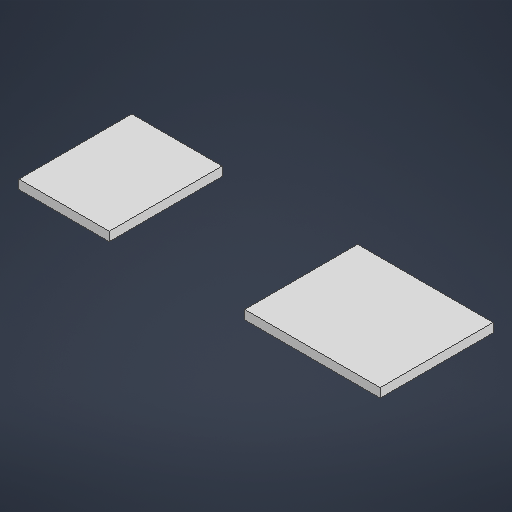
# Autodesk Inventor part: Krytka
Saved by Autodesk Inventor 2026.2 (Build 302298000, 298)
## iProperties
Created: 2026-04-16
Part Number: Krytka
Material: Všeobecné
Document SubType Name: Modeling
Designer: cerna
Density: 1 g/cm^3
Appearance: Výchozí
Author: cerna
Autodesk Inventor part; units mm, degrees
ref_plane "YZ Plane" through (0, 0, 0) normal (1, 0, 0) x (0, 1, 0)
ref_plane "XZ Plane" through (0, 0, 0) normal (0, 1, 0) x (-1, 0, 0)
ref_plane "XY Plane" through (0, 0, 0) normal (0, 0, 1) x (1, 0, 0)
sketch "Náčrt1" plane through (0, 0, 0) normal (0, 1, 0) x (-1, 0, 0)
  line L0 (0, -21.3939) -> (0, 14.3929) projected
  line L1 (-96, 0) -> (16, 0) projected
  line L2 (0, 9.2805) -> (-80, 9.2805)
  line L3 (-80, 9.2805) -> (-80, -15.7195)
  line L4 (-80, -15.7195) -> (0, -15.7195)
  line L5 (0, -15.7195) -> (0, 9.2805)
  line L6 (-20, 9.2805) -> (-20, -15.7195)
  line L7 (-50, 9.2805) -> (-50, -16.2815)
  point P0 (0, 0)
  point P1 (-50, -15.7195)
  point P2 (0, -15.7195)
  dimension "d0" = 25
  dimension "d1" = 80
  dimension "d2" = 20
  dimension "d3" = 30
  constraints: 12 end point, 4 point on line, 3 perpendicular, 2 parallel, 1 horizontal
  measures "d0" distance between parallel lines of L4 L2
  measures "d1" distance between parallel lines of L3 L0
  measures "d2" distance between parallel lines of L6 L0
  measures "d3" distance between parallel lines of L7 L3
extrude "Vysunutí1" add sketch "Náčrt1" along normal blind 2 contours L4 L6 L1 L0 | L1 L6 L2 L0 | L4 L3 L1 L7 | L1 L3 L2 L7
